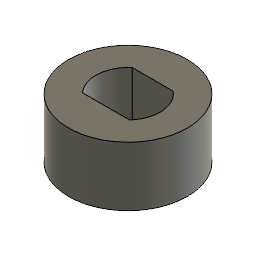
spacer (Autodesk Fusion 360 design; units mm, degrees)
part number: 2026-03-19-16-02-24-374
Autodesk Fusion 360 part; units mm, degrees
sketch "Sketch1" plane through (0, 0, 0) normal (0, 1, 0) x (1, 0, 0)
  circle A0 centre (0, 0) radius 2.7
  line L0 (1.9665, 0) -> (1.9665, -1.85)
  line L1 (1.9665, -1.85) -> (0, -1.85)
  line L2 (1.9665, -1.85) -> (-1.7335, -1.85)
  line L3 (-1.7335, -1.85) -> (-1.7335, 2.083)
  line L4 (-1.7335, 2.083) -> (1.9665, 2.083)
  line L5 (1.9665, 2.083) -> (1.9665, -1.85)
  line L6 (1.9665, -1.85) -> (-3, -1.85)
  line L7 (-3, -1.85) -> (4.3738, -1.85)
  line L8 (1.9665, 2.083) -> (-2.5, 2.083)
  dimension "d1" = 5.4
  dimension "d2" = 1.9665
  dimension "d3" = 1.85
  dimension "d4" = 3.7
  dimension "d5" = 3.933
  constraint coincident A0.centre origin
  constraint vertical L0
  constraint horizontal L1
  constraint horizontal L2
  constraint vertical L3
  constraint horizontal L4
  constraint vertical L5
  constraint perpendicular L3 L6
  constraint parallel L6 L7
  constraint perpendicular L5 L8
  measures "d1" diameter of A0
  measures "d2" distance of A0.centre L0.start
  measures "d3" distance of A0.centre L1.end
  measures "d4" distance of L0.end L2.end
  measures "d5" distance of L0.end L4.end
extrude "Extrude1" add sketch "Sketch1" along normal blind 1 contours A0 L0 L5 | A0 L0 L1 L2 L3 L4 L5 L6 L7 L8 | A0 L3 L6 L7 makes body 1
sketch "Sketch2" plane through (0, 1, 0) normal (0, 1, 0) x (-1, 0, 0)
  arc A0 (-1.9666, 1.85) -> (-1.7179, -2.083) centre (0, 0) ccw
  line L0 (-1.7179, -2.083) -> (1.7179, -2.083)
  arc A1 (1.7179, -2.083) -> (1.9666, 1.85) centre (0, 0) ccw
  line L1 (1.9666, 1.85) -> (-1.9666, 1.85)
  circle A2 centre (0, 0) radius 5
  dimension "d8" = 10
  constraint coincident A0.centre A1.centre
  measures "d8" diameter of A2
extrude "Extrude2" add sketch "Sketch2" along normal blind 4 and the other way blind 1 separate body makes body 2
combine "Combine1" operation cut target body 2 tool bodies 1
